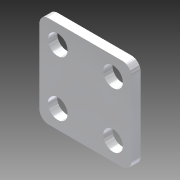
# Autodesk Inventor part: V5 Spacer Plate
Saved by Autodesk Inventor 2014 SP1 (Build 180222100, 222)
## iProperties
Created: 2012-02-04
Part Number: V5 Spacer Plate
Material: Aluminum-6061
Document SubType Name: Modeling
Designer: Moses
Mass: 7.36523 g
Surface Area: 23.6748 cm^2
Volume: 2.7178 cm^3
Density: 2.71 g/cm^3
Appearance: Aluminum - Polished
Author: Moses
Autodesk Inventor part; units mm, degrees
ref_plane "YZ Plane" through (0, 0, 0) normal (1, 0, 0) x (0, 1, 0)
ref_plane "XZ Plane" through (0, 0, 0) normal (0, 1, 0) x (-1, 0, 0)
ref_plane "XY Plane" through (0, 0, 0) normal (0, 0, 1) x (1, 0, 0)
sketch "Sketch1" plane through (0, 0, 0) normal (0, 0, 1) x (1, 0, 0)
  line L0 (0, 0) -> (0, 31.75)
  line L1 (0, 31.75) -> (31.75, 31.75)
  line L2 (31.75, 31.75) -> (31.75, 0)
  line L3 (31.75, 0) -> (0, 0)
  circle A0 centre (6.35, 25.4) radius 3.3782
  circle A1 centre (25.4, 25.4) radius 3.3782
  circle A2 centre (6.35, 6.35) radius 3.3782
  circle A3 centre (25.4, 6.35) radius 3.3782
  line L4 (15.875, 31.75) -> (15.875, 0) construction
  line L5 (0, 15.875) -> (31.75, 15.875) construction
  line L6 (25.4, 25.4) -> (25.4, 6.35) construction
  line L7 (6.35, 25.4) -> (25.4, 25.4) construction
  point P0 (25.4, 15.875)
  point P1 (15.875, 25.4)
  dimension "d0" = 31.75
  dimension "d1" = 31.75
  dimension "d2" = 6.7564
  dimension "d5" = 19.05
  dimension "d8" = 19.05
  constraints: 16 end point, 6 midpoint, 5 perpendicular, 4 centre point, 2 point on line, 2 vertical, 1 horizontal, 6 other
  measures "d0" distance of L0.start L0.end
  measures "d1" distance of L0.end L1.end
  measures "d2" diameter of A0
  measures "d5" distance of L7.start L6.start
  measures "d8" distance of L7.start A2.centre
extrude "Extrusion1" add sketch "Sketch1" along normal blind 3.175
fillet "Fillet1" radius 3.175 4 edges at (31.75, 31.75, 1.5875) (31.75, 0, 1.5875) (0, 31.75, 1.5875) (0, 0, 1.5875)
body "Solid1"
